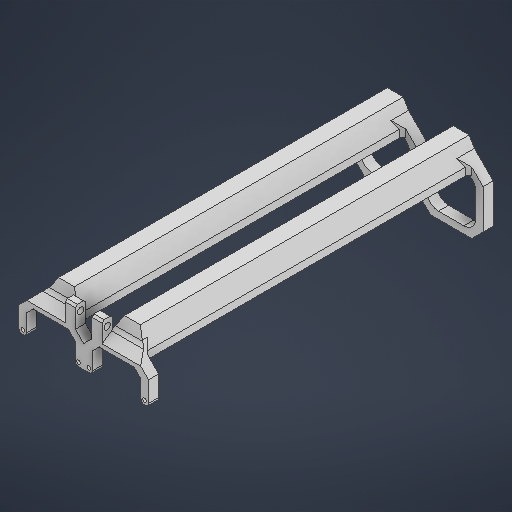
# Autodesk Inventor part: BatteryHolderBrackete
Saved by Autodesk Inventor 2026.1 (Build 301233000, 233)
## iProperties
Created: 2026-06-27
Part Number: BatteryHolderBrackete
Material: Generic
Document SubType Name: Modeling
Designer: Brynjar
Density: 1 g/cm^3
Appearance: Default
Author: Brynjar
Autodesk Inventor part; units mm, degrees
ref_plane "YZ Plane" through (0, 0, 0) normal (1, 0, 0) x (0, 1, 0)
ref_plane "XZ Plane" through (0, 0, 0) normal (0, 1, 0) x (-1, 0, 0)
ref_plane "XY Plane" through (0, 0, 0) normal (0, 0, 1) x (1, 0, 0)
derived "BatteryHolder.ipt"
sketch "Sketch1" plane through (0, 0, 0) normal (0, 0, 1) x (1, 0, 0)
  line L0 (-20.5, 11.5) -> (-20.5, -11.5)
  line L1 (-12.5, -19.5) -> (12.5, -19.5)
  line L2 (20.5, -11.5) -> (20.5, 11.5)
  line L3 (12.5, 19.5) -> (-12.5, 19.5)
  arc A0 (-12.5, 19.5) -> (-20.5, 11.5) centre (-12.5, 11.5) ccw
  arc A1 (20.5, 11.5) -> (12.5, 19.5) centre (12.5, 11.5) ccw
  arc A2 (12.5, -19.5) -> (20.5, -11.5) centre (12.5, -11.5) ccw
  arc A3 (-20.5, -11.5) -> (-12.5, -19.5) centre (-12.5, -11.5) ccw
  line L4 (0, 19.5) -> (0, -19.5) construction
  line L5 (-12.5, 22.5) -> (12.5, 22.5)
  arc A4 (23.5, 11.5) -> (12.5, 22.5) centre (12.5, 11.5) ccw
  line L6 (23.5, 11.5) -> (23.5, -11.5)
  arc A5 (12.5, -22.5) -> (23.5, -11.5) centre (12.5, -11.5) ccw
  line L7 (12.5, -22.5) -> (-12.5, -22.5)
  arc A6 (-23.5, -11.5) -> (-12.5, -22.5) centre (-12.5, -11.5) ccw
  line L8 (-23.5, -11.5) -> (-23.5, 11.5)
  arc A7 (-12.5, 22.5) -> (-23.5, 11.5) centre (-12.5, 11.5) ccw
  point P0 (0, 0)
  point P1 (0, 0)
sketch "Sketch3" plane through (0, 0, 370) normal (0, 0, 1) x (1, 0, 0)
  line L0 (-23.5, -11.5) -> (-23.5, 11.5) construction
  arc A0 (-12.5, 22.5) -> (-23.5, 11.5) centre (-12.5, 11.5) ccw construction
  line L1 (-12.5, 22.5) -> (12.5, 22.5) construction
  arc A1 (23.5, 11.5) -> (12.5, 22.5) centre (12.5, 11.5) ccw construction
  line L2 (23.5, 11.5) -> (23.5, -11.5) construction
  circle A2 centre (-27.5, 0) radius 1.8
  line L3 (-31.5, -2.75) -> (-31.5, 2.75) construction
  line L4 (-27.5, 0) -> (-31.5, 0) construction
  line L5 (-24, -0.8158) -> (-24, 16.2635)
  line L6 (-31.5, 19.3701) -> (-31.5, -0.8158)
  arc A3 (-27.1842, -4) -> (-24, -0.8158) centre (-27.1842, -0.8158) ccw
  arc A4 (-31.5, -0.8158) -> (-28.3158, -4) centre (-28.3158, -0.8158) ccw
  line L7 (-28.3158, -4) -> (-27.1842, -4)
  line L8 (-27.5, 0) -> (-27.5, -4) construction
  line L9 (-27.5, 0) -> (-24.9326, -3.0674) construction
  line L10 (17.2635, 23) -> (-17.2635, 23)
  line L11 (-24, -0.8158) -> (-23.5, -0.8158) construction
  line L12 (0, 22.5) -> (0, 23) construction
  line L13 (-17.2635, 23) -> (-24, 16.2635)
  line L14 (-31.5, 19.3701) -> (-20.3701, 30.5)
  line L15 (17.2635, 23) -> (24, 16.2635)
  line L16 (24, 16.2635) -> (24, -0.8158)
  line L17 (24, -0.8158) -> (23.5, -0.8158) construction
  line L18 (-20.3701, 30.5) -> (20.3701, 30.5)
  line L19 (-20.6317, 19.6317) -> (-25.935, 24.935) construction
  line L20 (-24, 16.2635) -> (-31.5, 16.2635) construction
  line L21 (-17.2635, 23) -> (-17.2635, 30.5) construction
  line L22 (-20.6317, 19.6317) -> (-20.2782, 19.2782) construction
  arc A5 (24, -0.8158) -> (27.1842, -4) centre (27.1842, -0.8158) ccw
  circle A6 centre (27.5, 0) radius 1.8
  line L23 (-27.5, 0) -> (-23.5, 0) construction
  line L24 (23.5, 0) -> (27.5, 0) construction
  line L25 (27.5, 0) -> (31.5, 0) construction
  line L26 (32.5, -4) -> (32.5, 0) construction
  line L27 (20.3701, 30.5) -> (32.5, 18.3701)
  line L28 (27.1842, -4) -> (32.5, -4)
  line L29 (20.6317, 19.6317) -> (25.935, 24.935) construction
  circle A7 centre (92.5, 0) radius 1.8
  line L30 (89, -0.8158) -> (89, 16.2635)
  line L31 (96.5, 19.3701) -> (96.5, -0.8158)
  arc A8 (89, -0.8158) -> (92.1842, -4) centre (92.1842, -0.8158) ccw
  arc A9 (93.3158, -4) -> (96.5, -0.8158) centre (93.3158, -0.8158) ccw
  line L32 (93.3158, -4) -> (92.1842, -4)
  line L33 (47.7365, 23) -> (82.2635, 23)
  line L34 (82.2635, 23) -> (89, 16.2635)
  line L35 (96.5, 19.3701) -> (85.3701, 30.5)
  line L36 (47.7365, 23) -> (41, 16.2635)
  line L37 (41, 16.2635) -> (41, -0.8158)
  line L38 (85.3701, 30.5) -> (44.6299, 30.5)
  arc A10 (37.8158, -4) -> (41, -0.8158) centre (37.8158, -0.8158) ccw
  circle A11 centre (37.5, 0) radius 1.8
  line L39 (44.6299, 30.5) -> (32.5, 18.3701)
  line L40 (37.8158, -4) -> (32.5, -4)
  line L41 (32.5, 0) -> (31.5, 0) construction
  point P0 (0, 0)
  dimension "d2" = 3.6
  dimension "d4" = 0.5
  dimension "d7" = 1
  constraints: 76 end point, 18 symmetric about line, 14 point on circle, 12 perpendicular, 11 equal length, 10 centre point, 8 midpoint, 8 point on line, 7 horizontal, 6 tangent, 3 equal radius, 3 vertical, 1 coincident, 1 line through centre, 1 parallel, 5 other
  measures "d2" diameter of A2
  measures "d4" distance of L5.start L11.end
  measures "d7" distance of L26.end L25.end
extrude "Extrusion1" add sketch "Sketch3" against normal blind 10
sketch "Sketch4" plane through (0, 0, 370) normal (0, 0, 1) x (1, 0, 0)
  line L0 (32.5, 18.3701) -> (32.5, 46.8) construction
  line L1 (32.5, 46.8) -> (40.65, 46.8) construction
  line L2 (40.65, 46.8) -> (40.65, 26.5201)
  line L3 (32.5, 46.8) -> (24.35, 46.8) construction
  line L4 (24.35, 46.8) -> (24.35, 26.5201)
  line L5 (44.6299, 30.5) -> (32.5, 18.3701) projected
  line L6 (32.5, 18.3701) -> (20.3701, 30.5) projected
  line L7 (14.35, 46.8) -> (14.35, 30.5)
  line L8 (50.65, 46.8) -> (50.65, 30.5)
  line L9 (24.35, 46.8) -> (14.35, 46.8)
  line L10 (40.65, 46.8) -> (50.65, 46.8)
  line L11 (85.3701, 30.5) -> (44.6299, 30.5) projected
  line L12 (20.3701, 30.5) -> (-20.3701, 30.5) projected
  line L13 (40.65, 38.65) -> (50.65, 38.65) construction
  line L14 (45.65, 41.8) -> (45.65, 35.5) construction
  line L15 (45.65, 41.8) -> (45.65, 46.8) construction
  line L16 (45.65, 35.5) -> (45.65, 30.5) construction
  point P0 (0, 0)
  point P1 (45.65, 38.65)
  dimension "d9" = 10
  dimension "d10" = 16.3
  dimension "d12" = 6.3
  dimension "d15" = 5
  constraints: 26 end point, 7 point on line, 4 collinear, 4 midpoint, 4 vertical, 3 horizontal, 3 perpendicular
  measures "d9" distance of L1.end L8.start
  measures "d10" distance between parallel lines of L4 L2
  measures "d12" distance of L14.start L14.end
  measures "d15" distance of L14.start L15.end
extrude "Extrusion2" add sketch "Sketch4" against normal up to surface (10 mm away)
sketch "Sketch6" plane through (50.65, 30.5, 370) normal (1, 0, 0) x (0, 0, -1)
  circle A0 centre (5, 9.3) radius 3.15
  line L0 (10, 0) -> (10, 16.3) construction
  line L1 (0, 0) -> (0, 16.3) construction
  line L2 (0, 9.3) -> (5, 9.3) construction
  line L3 (5, 9.3) -> (5, 16.3) construction
  line L4 (0, 16.3) -> (10, 16.3) construction
  line L5 (5, 9.3) -> (10, 9.3) construction
  point P0 (370, -30.5)
  point P1 (5, 9.3)
  dimension "d18" = 6.3
  dimension "d22" = 7
  constraints: 6 end point, 3 perpendicular, 2 coincident, 2 point on line, 1 centre point, 1 midpoint
  measures "d18" diameter of A0
  measures "d22" distance of L2.end L3.end
extrude "Extrusion3" cut sketch "Sketch6" against normal through all
chamfer "Chamfer1" distance 2 angle 45 4 edges at (45.65, 46.8, 370) (45.65, 46.8, 360) (19.35, 46.8, 370) (19.35, 46.8, 360)
sketch "Sketch7" plane through (0, 0, 360) normal (0, 0, -1) x (-1, 0, 0)
  line L0 (-82.2635, 23) -> (-47.7365, 23) projected
  line L1 (-50.65, 30.5) -> (-85.3701, 30.5) projected
  line L2 (20.3701, 30.5) -> (-14.35, 30.5) projected
  line L3 (-17.2635, 23) -> (17.2635, 23) projected
  line L4 (-82.2635, 23) -> (-82.2635, 30.5)
  line L5 (-47.7365, 23) -> (-82.2635, 23) projected
  line L6 (-47.7365, 23) -> (-47.7365, 30.5)
  line L7 (-47.7365, 30.5) -> (-50.65, 30.5)
  line L8 (-17.2635, 23) -> (-17.2635, 30.5)
  line L9 (-17.2635, 30.5) -> (-14.35, 30.5)
  line L10 (17.2635, 23) -> (17.2635, 30.5)
  point P0 (0, 0)
  constraints: 12 end point, 5 perpendicular, 3 point on line, 1 vertical
extrude "Extrusion4" add sketch "Sketch7" along normal blind 320
sketch "Sketch8" plane through (0, 0, 40) normal (0, 0, -1) x (-1, 0, 0)
  line L0 (12.5, 22.5) -> (-12.5, 22.5) construction
  arc A0 (-12.5, 22.5) -> (-23.5, 11.5) centre (-12.5, 11.5) ccw construction
  arc A1 (23.5, 11.5) -> (12.5, 22.5) centre (12.5, 11.5) ccw construction
  line L1 (23.5, -11.5) -> (23.5, 11.5) construction
  arc A2 (12.5, -22.5) -> (23.5, -11.5) centre (12.5, -11.5) ccw construction
  line L2 (-12.5, -22.5) -> (12.5, -22.5) construction
  arc A3 (-23.5, -11.5) -> (-12.5, -22.5) centre (-12.5, -11.5) ccw construction
  line L3 (-23.5, 11.5) -> (-23.5, -11.5) construction
  line L4 (12.5, 23.5) -> (-12.5, 23.5) construction
  arc A4 (-12.5, 23.5) -> (-24.5, 11.5) centre (-12.5, 11.5) ccw
  line L5 (-24.5, 11.5) -> (-24.5, -11.5)
  arc A5 (-24.5, -11.5) -> (-12.5, -23.5) centre (-12.5, -11.5) ccw
  line L6 (-12.5, -23.5) -> (12.5, -23.5)
  arc A6 (12.5, -23.5) -> (24.5, -11.5) centre (12.5, -11.5) ccw
  line L7 (24.5, -11.5) -> (24.5, 11.5)
  arc A7 (24.5, 11.5) -> (12.5, 23.5) centre (12.5, 11.5) ccw
  line L8 (20.3701, 30.5) -> (-20.3701, 30.5) projected
  line L9 (31.5, 19.3701) -> (20.3701, 30.5) projected
  line L10 (-20.3701, 30.5) -> (-32.5, 18.3701) projected
  line L11 (31.5, 19.3701) -> (31.5, -19.3701)
  line L12 (31.5, -19.3701) -> (20.3701, -30.5)
  line L13 (20.3701, -30.5) -> (-20.3701, -30.5)
  line L14 (-20.3701, -30.5) -> (-32.5, -18.3701)
  line L15 (-32.5, -18.3701) -> (-32.5, 18.3701) construction
  line L16 (0, -23.5) -> (0, -30.5) construction
  line L17 (0, 23.5) -> (0, 30.5) construction
  line L18 (-77.5, 23.5) -> (-52.5, 23.5) construction
  arc A8 (-40.5, 11.5) -> (-52.5, 23.5) centre (-52.5, 11.5) ccw
  line L19 (-40.5, 11.5) -> (-40.5, -11.5)
  arc A9 (-52.5, -23.5) -> (-40.5, -11.5) centre (-52.5, -11.5) ccw
  line L20 (-52.5, -23.5) -> (-77.5, -23.5)
  arc A10 (-89.5, -11.5) -> (-77.5, -23.5) centre (-77.5, -11.5) ccw
  line L21 (-89.5, -11.5) -> (-89.5, 11.5)
  arc A11 (-77.5, 23.5) -> (-89.5, 11.5) centre (-77.5, 11.5) ccw
  line L22 (-85.3701, 30.5) -> (-44.6299, 30.5)
  line L23 (-96.5, 19.3701) -> (-85.3701, 30.5)
  line L24 (-44.6299, 30.5) -> (-32.5, 18.3701)
  line L25 (-96.5, 19.3701) -> (-96.5, -19.3701)
  line L26 (-96.5, -19.3701) -> (-85.3701, -30.5)
  line L27 (-85.3701, -30.5) -> (-44.6299, -30.5)
  line L28 (-44.6299, -30.5) -> (-32.5, -18.3701)
  line L29 (-82.2635, 23) -> (-47.7365, 23) projected
  line L30 (-17.2635, 23) -> (17.2635, 23) projected
  point P0 (0, 0)
  point P1 (-15.9278, 23)
  point P2 (15.9278, 23)
  point P3 (-80.9278, 23)
  point P4 (-49.0722, 23)
  dimension "d27" = 1
  constraints: 44 end point, 18 symmetric about line, 16 point on circle, 8 centre point, 4 midpoint, 3 equal length, 3 perpendicular, 2 vertical, 11 other
  measures "d27" distance between parallel lines of L3 L5
extrude "Extrusion5" add sketch "Sketch8" along normal blind 10
chamfer "Chamfer3" distance 3.11 angle 45 8 edges at (-17.2635, 26.75, 360) (17.2635, 26.75, 360) (17.2635, 26.75, 40) (-17.2635, 26.75, 40) (47.7365, 26.75, 40) (82.2635, 26.75, 40) (82.2635, 26.75, 360) (47.7365, 26.75, 360)
sketch "Sketch9" plane through (0, 0, 30) normal (0, 0, -1) x (-1, 0, 0)
  line L0 (-14.35, 46.8) -> (-24.35, 46.8) construction
  line L1 (7.8526, 46.8) -> (-7.8526, 46.8)
  line L2 (20.3701, 30.5) -> (-20.3701, 30.5) projected
  line L3 (-7.8526, 46.8) -> (-17.2635, 30.5)
  line L4 (7.8526, 46.8) -> (17.2635, 30.5)
  line L5 (0, 46.8) -> (0, 30.5) construction
  point P0 (0, 0)
  dimension "d49" = 60
  constraints: 8 end point, 2 midpoint, 1 collinear, 1 horizontal, 1 perpendicular
  measures "d49" angle of L2 L3
extrude "Extrusion6" add sketch "Sketch9" against normal up to surface (340 mm away)
ref_plane "Work Plane3" through (32.5, -0.8158, 370) normal (-1, 0, 0) x (0, 0, 1)
mirror "Mirror1" about plane through (32.5, -0.8158, 370) normal (-1, 0, 0) of "Extrusion6"
delete faces "Delete Face1" heal yes whole lump no faces at (-18.299, 30.5, 37.7045) (18.299, 30.5, 37.7045) (46.701, 30.5, 37.7045) (83.299, 30.5, 37.7045) (46.6999, 30.5, 358.9633) (18.3001, 30.5, 358.9633)
delete faces "Delete Face2" heal yes whole lump no faces at (83.299, 30.5, 362.2955) (-18.299, 30.5, 362.2955)
sketch "Sketch10" plane through (-31.5, -0.8158, 370) normal (-1, 0, 0) x (0, 0, 1)
  circle A0 centre (-5, 40.6158) radius 3.15 construction
  arc A1 (-9.3018, 34.4721) -> (-12.0477, 38.0506) centre (-5, 40.6158) ccw construction
  line L0 (-12.0477, 38.0506) -> (-15.5291, 47.6158)
  line L1 (-340, 47.6158) -> (0, 47.6158) projected
  line L2 (-9.3018, 34.4721) -> (0, 27.9589)
  line L3 (0, 38.6661) -> (0, 20.1858) projected
  arc A2 (-12.0477, 38.0506) -> (-9.3018, 34.4721) centre (-5, 40.6158) ccw
  line L4 (0, 38.6661) -> (0, 47.6158)
  line L5 (-13.11, 31.3158) -> (-326.89, 31.3158) projected
  point P0 (-370, 0.8158)
  point P1 (0, 47.6158)
  dimension "d50" = 15
  dimension "d51" = 55
  dimension "d52" = 20
  constraints: 6 end point, 4 point on circle, 2 centre point, 2 point on line, 2 tangent, 1 coincident, 1 perpendicular
  measures "d50" diameter of A1
  measures "d51" angle of L3 L2
  measures "d52" angle of L3 L0
extrude "Extrusion7" cut sketch "Sketch10" against normal up to surface (45.85 mm away)
mirror "Mirror2" about plane through (32.5, -0.8158, 370) normal (-1, 0, 0) of "Extrusion7"
sketch "Sketch5" plane through (0, 0, 370) normal (0, 0, 1) x (1, 0, 0)
  line L0 (-23.5, 11.5) -> (-23.5, -11.5) projected
  circle A0 centre (-27.5, 0) radius 1.7 projected
  circle A1 centre (-27.5, 0) radius 2.75 construction
  line L1 (-31.5, -2.75) -> (-31.5, 2.75) projected
  arc A2 (-31.5, -2.75) -> (-29.6787, -4.742) centre (-29.5, -2.75) ccw projected
  arc A3 (-29.6787, 4.742) -> (-31.5, 2.75) centre (-29.5, 2.75) ccw projected
  arc A4 (-23.5, -11.5) -> (-29.6787, -4.742) centre (-30.2852, -11.5) ccw projected
  arc A5 (-29.6787, 4.742) -> (-23.5, 11.5) centre (-30.2852, 11.5) ccw projected
  line L2 (-31.5, 2.75) -> (-27.5, 2.75) construction
  circle A6 centre (-27.5, 0) radius 4 construction
  point P0 (0, 0)
  point P1 (-23.5, 0)
  point P2 (-31.5, 0)
  constraints: 1 horizontal alignment, 1 vertical alignment
ref_plane "Work Plane2" through (0, 0, 370) normal (0, 0, 1) x (1, 0, 0)
body "Solid1"
